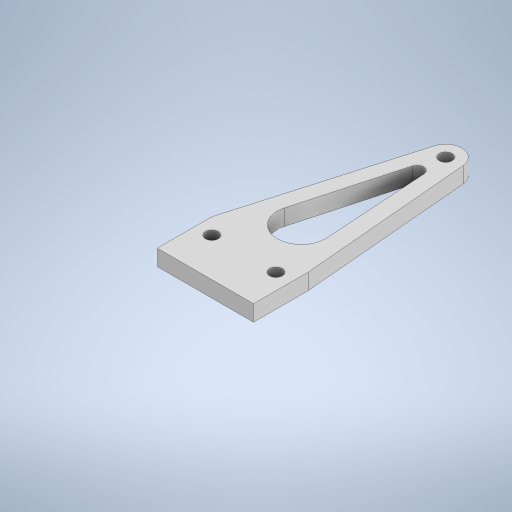
# Autodesk Inventor part: Pieza3
Saved by Autodesk Inventor 2024.3 (Build 283343000, 343)
## iProperties
Created: 2025-01-27
Part Number: Pieza3
Material: Genérico
Document SubType Name: Modeling
Designer: Jorge
Density: 1 g/cm^3
Appearance: Valor por defecto
Author: Jorge
Autodesk Inventor part; units mm, degrees
ref_plane "YZ Plane" through (0, 0, 0) normal (1, 0, 0) x (0, 1, 0)
ref_plane "XZ Plane" through (0, 0, 0) normal (0, 1, 0) x (-1, 0, 0)
ref_plane "XY Plane" through (0, 0, 0) normal (0, 0, 1) x (1, 0, 0)
sketch "Boceto1" plane through (0, 0, 0) normal (1, 0, 0) x (0, 1, 0)
  point P0 (0, 0)
sketch "Boceto2" plane through (0, 0, 0) normal (0, 1, 0) x (-1, 0, 0)
  line L0 (0, 0) -> (30, 0)
  line L1 (30, 0) -> (30, -60)
  line L2 (30, -60) -> (0, -60)
  line L3 (0, -60) -> (0, 0)
  circle A0 centre (25, -5) radius 2
  line L4 (30, -30) -> (0, -30) construction
  circle A1 centre (25, -55) radius 2
  line L5 (15, 0) -> (15, -60) construction
  circle A2 centre (5, -5) radius 2
  circle A3 centre (5, -55) radius 2
  line L6 (0, -60) -> (4.6345, -112.9721)
  line L7 (0, -60) -> (53.1744, -60) construction
  line L8 (30, -60) -> (14.4189, -113.9242)
  line L9 (0, 0) -> (4.6345, 52.9721)
  line L10 (30, 0) -> (14.4189, 53.9242)
  arc A4 (14.4189, 53.9242) -> (4.6345, 52.9721) centre (9.6154, 52.5363) ccw
  arc A5 (4.6345, -112.9721) -> (14.4189, -113.9242) centre (9.6154, -112.5363) ccw
  circle A6 centre (9.6154, -112.5363) radius 2
  circle A7 centre (9.6154, 52.5363) radius 2
  line L11 (15, -60) -> (9.1311, -117.5128) construction
  line L12 (1.0267, -71.7351) -> (26.6092, -71.7351) construction
  arc A8 (21.0465, -73.7346) -> (6.3341, -72.2264) centre (13.818, -71.7351) ccw
  arc A9 (8.462, -104.6439) -> (12.3853, -105.0461) centre (10.4577, -104.5129) ccw
  line L13 (21.0465, -73.7346) -> (12.3853, -105.0461)
  line L14 (6.3018, -71.7351) -> (8.462, -104.6439)
  arc A10 (6.3341, 12.2264) -> (21.0465, 13.7346) centre (13.818, 11.7351) ccw
  arc A11 (12.3853, 45.0461) -> (8.462, 44.6439) centre (10.4577, 44.5129) ccw
  line L15 (21.0465, 13.7346) -> (12.3853, 45.0461)
  line L16 (6.3018, 11.7351) -> (8.462, 44.6439)
  point P0 (6.9725, -139.6956)
  point P1 (6.9725, 79.6956)
  dimension "d0" = 30
  dimension "d1" = 60
  dimension "d2" = 4
  dimension "d4" = 5
  dimension "d5" = 5
  dimension "d6" = 80
  dimension "d7" = 85
  dimension "d8" = 5
  dimension "d9" = 4
  dimension "d10" = 4
  dimension "d11" = 15
  dimension "d12" = 4
  dimension "d13" = 0.654
  constraints: 34 end point, 13 point on circle, 12 centre point, 11 symmetric about line, 10 point on line, 8 tangent, 5 midpoint, 3 horizontal, 2 coincident, 2 parallel, 1 equal length, 1 equal radius, 1 perpendicular, 5 other
  measures "d0" distance of L1.end L2.end
  measures "d1" distance of L0.end L1.end
  measures "d2" diameter of A0
  measures "d4" distance from line of A0.centre L1
  measures "d5" distance from line of A0.centre L0
  measures "d6" distance of L2.end point (6.972, -139.696)
  measures "d7" angle of L6 L7
  measures "d8" radius of A4
  measures "d9" diameter of A6
  measures "d10" diameter of A7
  measures "d11" diameter of A8
  measures "d12" diameter of A9
  measures "d13" angle of L8 L13
extrude "Extrusión1" add sketch "Boceto2" along normal blind 5
sketch "Boceto3" plane through (0, 5, 0) normal (0, 1, 0) x (1, 0, 0)
  point P0 (0, 0)
fillet "Empalme1" radius 10 2 edges at (-30, 2.5, 0) (-30, 2.5, -60)
sketch "Boceto5" plane through (0, 5, 0) normal (0, 1, 0) x (1, 0, 0)
  circle A0 centre (-5, 55) radius 2 construction
  line L0 (-5, 53) -> (-5, 43) construction
  line L1 (6.8466, 43) -> (-33.4625, 43)
  line L2 (-33.4625, 43) -> (-33.4625, -74.7352)
  line L3 (-33.4625, -74.7352) -> (6.8466, -74.7352)
  line L4 (6.8466, -74.7352) -> (6.8466, 43)
  point P0 (0, 0)
  dimension "d18" = 10
  constraints: 10 end point, 2 parallel, 1 horizontal, 1 perpendicular, 1 vertical, 1 vertical alignment, 1 other
  measures "d18" distance of L0.start L0.end
extrude "Extrusión2" cut sketch "Boceto5" against normal blind 10
